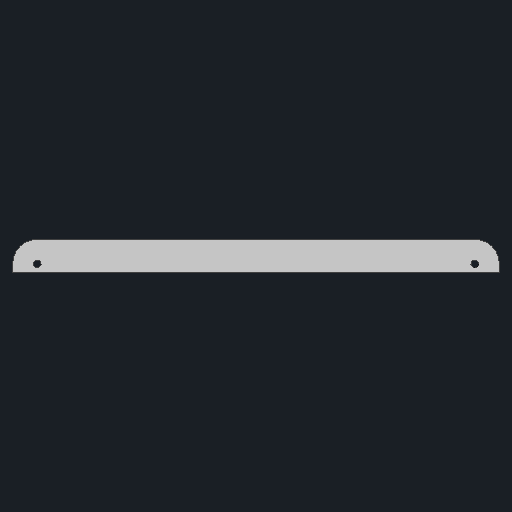
# Autodesk Inventor part: io_fix
Saved by Autodesk Inventor 2026 (Build 300175000, 175)
## iProperties
Created: 2026-02-13
Part Number: io_fix
Material: 一般
Document SubType Name: Modeling
Designer: numai
Density: 1 g/cm^3
Appearance: 既定
Author: numai
Autodesk Inventor part; units mm, degrees
ref_plane "YZ Plane" through (0, 0, 0) normal (1, 0, 0) x (0, 1, 0)
ref_plane "XZ Plane" through (0, 0, 0) normal (0, 1, 0) x (-1, 0, 0)
ref_plane "XY Plane" through (0, 0, 0) normal (0, 0, 1) x (1, 0, 0)
sketch "スケッチ1" plane through (0, 0, 0) normal (0, 0, 1) x (1, 0, 0)
  line L0 (-1.1, 1.1) -> (-1.1, 157.58) construction
  line L1 (42.18, 0) -> (0, 0) construction
  line L2 (43.28, 157.58) -> (43.28, 1.1) construction
  line L3 (0, 158.68) -> (42.18, 158.68) construction
  line L4 (43.28, 0) -> (-1.1, 0)
  line L5 (-1.1, 0) -> (-1.1, 158.68)
  line L6 (-1.1, 158.68) -> (43.28, 158.68)
  line L7 (43.28, 158.68) -> (43.28, 0)
  line L8 (49.121, 378.1158) -> (49.121, -108.9393) construction
  line L9 (49.121, -20) -> (-6.941, -20)
  line L10 (-6.941, -20) -> (-6.941, 178.68)
  line L11 (-6.941, 178.68) -> (49.121, 178.68)
  line L12 (49.121, 178.68) -> (49.121, -20)
  dimension "d0" = 20
  dimension "d1" = 20
  dimension "d2" = 5.841
  dimension "d15" = 5.841
  constraints: 18 end point, 5 point on line, 4 parallel, 2 horizontal, 2 perpendicular, 1 vertical, 2 other
  measures "d0" distance between parallel lines of L1 L9
  measures "d1" distance between parallel lines of L11 L3
  measures "d2" distance between parallel lines of L10 L0
  measures "d15" distance between parallel lines of L8 L2
extrude "押し出し1" add sketch "スケッチ1" along normal blind 13.64
sketch "スケッチ2" plane through (-6.941, -20, 0) normal (-1, 0, 0) x (0, 0, 1)
  circle A0 centre (3.64, 10) radius 1.6 projected
  circle A1 centre (3.64, 188.68) radius 1.6 projected
  point P0 (0, 20)
extrude "押し出し2" cut sketch "スケッチ2" against normal through all
fillet "フィレット1" radius 10 2 edges at (21.09, 178.68, 13.64) (21.09, -20, 13.64)
sketch "スケッチ3" plane through (-6.941, -20, 0) normal (-1, 0, 0) x (0, 0, 1)
  circle A0 centre (3.64, 188.68) radius 1.6 construction
  circle A1 centre (3.64, 10) radius 1.6 construction
  circle A2 centre (3.64, 188.68) radius 1.6 projected
  circle A3 centre (3.64, 188.68) radius 6
  circle A4 centre (3.64, 10) radius 6
  point P0 (0, 20)
  dimension "d8" = 12
  constraints: 2 centre point, 2 coincident, 1 equal radius
  measures "d8" diameter of A3
extrude "押し出し3" cut sketch "スケッチ3" against normal blind 39.062
fillet "フィレット2" [suppressed]
fillet "フィレット3" radius 10 2 edges at (21.09, 0, 13.64) (21.09, 158.68, 13.64)
sketch "スケッチ4" plane through (-6.941, -10, 13.64) normal (-1, 0, 0) x (0, 0, 1)
  line L0 (-13.64, -4.7697) -> (-13.64, -10) projected
  line L1 (-13.64, 173.9103) -> (-13.64, 4.7697) projected
  arc A0 (-13.64, -4.7697) -> (-13.64, 4.7697) centre (-10, 0) ccw projected
  line L2 (-13.64, 188.68) -> (-13.64, 183.4497) projected
  arc A1 (-13.64, 173.9103) -> (-13.64, 183.4497) centre (-10, 178.68) ccw projected
  line L3 (-10, -6) -> (-13.64, -6)
  line L4 (-10, 6) -> (-13.64, 6)
  line L5 (-10, 172.68) -> (-13.64, 172.68)
  line L6 (-10, 184.68) -> (-13.64, 184.68)
  point P0 (-13.64, 10)
  constraints: 8 end point, 4 point on circle, 4 point on line, 4 tangent, 2 perpendicular, 1 horizontal, 1 parallel
extrude "押し出し4" cut sketch "スケッチ4" against normal up to surface (39.062 mm away)
equation "\"d1\" = d0"
equation "\"d2\" = d15"
